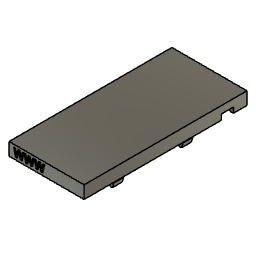
Attenuator top v9 (Autodesk Fusion 360 design; units mm, degrees)
Autodesk Fusion 360 part; units mm, degrees
sketch "Sketch1" plane through (0, 0, 0) normal (0, 0, 1) x (1, 0, 0)
  line L0 (-38.1, 55.88) -> (5.588, 55.88)
  line L1 (5.588, 55.88) -> (5.588, -46.1518)
  line L2 (5.588, -46.1518) -> (-38.1, -46.1518)
  line L3 (-38.1, -46.1518) -> (-38.1, 55.88)
  line L4 (-40.64, 57.785) -> (8.128, 57.785)
  line L5 (8.128, 57.785) -> (8.128, -48.0568)
  line L6 (8.128, -48.0568) -> (-40.64, -48.0568)
  line L7 (-40.64, -48.0568) -> (-40.64, 57.785)
  dimension "d1" = 43.688
  dimension "d2" = 102.0318
  dimension "d3" = 1.905
  dimension "d4" = 1.905
  dimension "d5" = 2.54
  dimension "d6" = 2.54
  constraint horizontal L0
  constraint vertical L1
  constraint horizontal L2
  constraint vertical L3
  constraint horizontal L4
  constraint vertical L5
  constraint horizontal L6
  constraint vertical L7
  measures "d1" distance of L0.start L0.end
  measures "d2" distance of L0.start L2.end
  measures "d3" distance of L0 L4
  measures "d4" distance of L2 L6
  measures "d5" distance of L3 L7
  measures "d6" distance of L1 L5
extrude "Extrude1" add sketch "Sketch1" along normal blind 1.905 contours L0 L1 L2 L3 | L4 L5 L6 L7
extrude "Extrude2" add sketch "Sketch1" against normal blind 6.35
sketch "Sketch3" plane through (-40.64, 0, 0) normal (-1, 0, 0) x (0, -1, 0)
  line L0 (48.0568, -6.35) -> (48.0568, 1.905)
  line L1 (48.0568, 1.905) -> (-57.785, 1.905)
  line L2 (-57.785, 1.905) -> (-57.785, -6.35)
  line L3 (-57.785, -6.35) -> (48.0568, -6.35)
  circle A0 centre (-45.085, -6.35) radius 3.175
  dimension "d15" = 6.35
  dimension "d16" = 12.7
  constraint coincident L3 A0.centre
  measures "d15" diameter of A0
  measures "d16" distance of L2.end A0.centre
extrude "Extrude4" cut sketch "Sketch3" against normal up to surface (2.54 mm away) contours L3 A0 picked at (-45.0059, -5.2946)
sketch "Sketch4" plane through (8.128, 0, 0) normal (1, 0, 0) x (0, 1, 0)
  line L0 (57.785, -6.35) -> (57.785, 1.905)
  line L1 (57.785, 1.905) -> (-48.0568, 1.905)
  line L2 (-48.0568, 1.905) -> (-48.0568, -6.35)
  line L3 (-48.0568, -6.35) -> (57.785, -6.35)
  line L4 (41.148, -2.85) -> (49.022, -2.85)
  line L5 (49.022, -2.85) -> (49.022, -6.35)
  line L6 (49.022, -6.35) -> (41.148, -6.35)
  line L7 (41.148, -6.35) -> (41.148, -2.85)
  dimension "d19" = 8.763
  dimension "d20" = 3.5
  dimension "d21" = 7.874
  constraint horizontal L4
  constraint vertical L5
  constraint horizontal L6
  constraint vertical L7
  constraint collinear L3 L6
  measures "d19" distance of L0 L5
  measures "d20" distance of L3 L4
  measures "d21" distance of L4.start L4.end
extrude "Extrude5" cut sketch "Sketch4" against normal up to surface (2.54 mm away) contours L3 L4 L5 L6 L7
sketch "Sketch5" plane through (-38.1, 0, 0) normal (1, 0, 0) x (0, 1, 0)
  arc A0 (48.26, -6.35) -> (41.91, -6.35) centre (45.085, -6.35) ccw
  line L0 (48.26, -6.35) -> (55.88, -6.35)
  line L1 (55.88, -6.35) -> (55.88, 0)
  line L2 (55.88, 0) -> (-46.1518, 0)
  line L3 (-46.1518, 0) -> (-46.1518, -6.35)
  line L4 (-46.1518, -6.35) -> (41.91, -6.35)
  line L5 (-27.1018, 0) -> (-20.7518, 0)
  line L6 (-20.7518, 0) -> (-20.7518, -11.43)
  line L7 (-20.7518, -11.43) -> (-27.1018, -11.43)
  line L8 (-27.1018, -11.43) -> (-27.1018, 0)
  line L9 (17.78, 0) -> (24.13, 0)
  line L10 (24.13, 0) -> (24.13, -11.43)
  line L11 (24.13, -11.43) -> (17.78, -11.43)
  line L12 (17.78, -11.43) -> (17.78, 0)
  dimension "d24" = 6.35
  dimension "d25" = 5.08
  dimension "d26" = 19.05
  dimension "d27" = 31.75
  constraint horizontal L5
  constraint vertical L6
  constraint horizontal L7
  constraint vertical L8
  constraint horizontal L9
  constraint vertical L10
  constraint horizontal L11
  constraint vertical L12
  constraint collinear L2 L5
  constraint collinear L2 L9
  constraint collinear L7 L11
  constraint equal L5 L9
  measures "d24" distance of L5.start L5.end
  measures "d25" distance of L4 L7
  measures "d26" distance of L3 L8
  measures "d27" distance of L1 L10
extrude "Extrude6" add sketch "Sketch5" along normal blind 1.905 contours L4 L10 L11 L12 | L2 L4 L9 L10 L12 | L4 L6 L7 L8 | L2 L4 L5 L6 L8
sketch "Sketch6" plane through (5.588, 0, 0) normal (-1, 0, 0) x (0, -1, 0)
  line L0 (-49.022, -6.35) -> (-49.022, -2.85)
  line L1 (-49.022, -2.85) -> (-41.148, -2.85)
  line L2 (-41.148, -2.85) -> (-41.148, -6.35)
  line L3 (-41.148, -6.35) -> (46.1518, -6.35)
  line L4 (46.1518, -6.35) -> (46.1518, 0)
  line L5 (46.1518, 0) -> (-55.88, 0)
  line L6 (-55.88, 0) -> (-55.88, -6.35)
  line L7 (-55.88, -6.35) -> (-49.022, -6.35)
  line L8 (-24.13, 0) -> (-17.78, 0)
  line L9 (-17.78, 0) -> (-17.78, -11.43)
  line L10 (-17.78, -11.43) -> (-24.13, -11.43)
  line L11 (-24.13, -11.43) -> (-24.13, 0)
  line L12 (20.7518, 0) -> (27.1018, 0)
  line L13 (27.1018, 0) -> (27.1018, -11.43)
  line L14 (27.1018, -11.43) -> (20.7518, -11.43)
  line L15 (20.7518, -11.43) -> (20.7518, 0)
  dimension "d30" = 5.08
  dimension "d31" = 6.35
  dimension "d32" = 19.05
  dimension "d33" = 31.75
  constraint horizontal L8
  constraint vertical L9
  constraint horizontal L10
  constraint vertical L11
  constraint coincident L5 L8.start
  constraint horizontal L12
  constraint vertical L13
  constraint horizontal L14
  constraint vertical L15
  constraint coincident L5 L12.start
  constraint equal L10 L14
  constraint collinear L10 L14
  measures "d30" distance of L3 L10
  measures "d31" distance of L8.start L8.end
  measures "d32" distance of L4 L13
  measures "d33" distance of L6 L11
extrude "Extrude7" add sketch "Sketch6" along normal blind 1.905 contours L3 L5 L8 L9 L11 | L3 L9 L10 L11 | L3 L5 L12 L13 L15 | L3 L13 L14 L15
sketch "Sketch7" plane through (0, 24.13, 0) normal (0, 1, 0) x (-1, 0, 0)
  line L0 (38.1, -6.35) -> (38.1, 0)
  line L1 (38.1, 0) -> (36.195, 0)
  line L2 (36.195, 0) -> (36.195, -11.43)
  line L3 (36.195, -11.43) -> (38.1, -11.43)
  line L4 (38.1, -11.43) -> (38.1, -6.35)
  line L5 (38.1, -11.43) -> (39.116, -8.255)
  line L6 (39.116, -8.255) -> (38.1, -8.255)
  line L7 (39.116, -8.255) -> (38.1, -6.35)
  dimension "d36" = 1.905
  dimension "d37" = 1.016
  constraint coincident L3.end L4.start
  constraint coincident L4 L6.end
  constraint perpendicular L4 L6
  constraint coincident L0.start L4.end
  measures "d36" distance of L0.start L6.end
  measures "d37" distance of L5.end L6.end
extrude "Extrude8" add sketch "Sketch7" against normal up to surface (6.35 mm away) contours L4 L6 L7 | L4 L5 L6
extrude "Extrude9" add sketch "Sketch7" against normal up to surface (6.35 mm away) from surface at -44.8818 contours L4 L6 L7 | L4 L5 L6
sketch "Sketch8" plane through (0, -27.1018, 0) normal (0, -1, 0) x (1, 0, 0)
  line L0 (5.588, -6.35) -> (5.588, 0)
  line L1 (5.588, 0) -> (3.683, 0)
  line L2 (3.683, 0) -> (3.683, -11.43)
  line L3 (3.683, -11.43) -> (5.588, -11.43)
  line L4 (5.588, -11.43) -> (5.588, -6.35)
  line L5 (5.588, -11.43) -> (6.604, -8.255)
  line L6 (6.604, -8.255) -> (5.588, -8.255)
  line L7 (6.604, -8.255) -> (5.588, -6.35)
  dimension "d43" = 1.016
  dimension "d44" = 1.905
  constraint coincident L3.end L4.start
  constraint coincident L4 L6.end
  constraint perpendicular L4 L6
  constraint coincident L0.start L4.end
  measures "d43" distance of L5.end L6.end
  measures "d44" distance of L0.start L6.end
extrude "Extrude10" add sketch "Sketch8" against normal blind 6.35 contours L4 L6 L7 | L4 L5 L6
extrude "Extrude11" add sketch "Sketch8" against normal up to surface (6.35 mm away) from surface at -44.8818 contours L4 L6 L7 | L4 L5 L6
sketch "Sketch9" plane through (0, -48.0568, 0) normal (0, -1, 0) x (1, 0, 0)
  line L0 (-40.64, -6.35) -> (8.128, -6.35)
  line L1 (8.128, -6.35) -> (8.128, 1.905)
  line L2 (8.128, 1.905) -> (-40.64, 1.905)
  line L3 (-40.64, 1.905) -> (-40.64, -6.35)
  line L4 (-40.64, -6.35) -> (-14.5034, -6.35) construction
  line L5 (-14.5034, -6.35) -> (-14.5034, 1.905) construction
  line L6 (-14.5034, 1.905) -> (-40.64, 1.905) construction
  line L7 (-40.64, 1.905) -> (-40.64, -6.35) construction
  dimension "d53" = 5.08
  dimension "d54" = 26.1366
  text T0 "WWW" font "Arial" height 5.08 bold align centre middle in box 26.1366 x 8.255 at (-40.64, -6.35) x (1, 0) y (0, 1) spacing 1 kerned
  constraint coincident L0.start
  constraint coincident L2.end
  measures "d54" distance of L2.end
extrude "Extrude12" cut sketch "Sketch9" against normal blind 1.016 text T0
